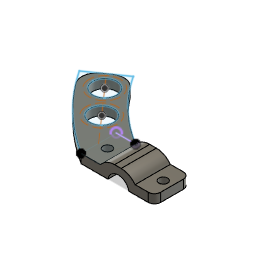
R1200GS Motorbike mirror button mount v3 (Autodesk Fusion 360 design; units mm, degrees)
Autodesk Fusion 360 part; units mm, degrees
sketch "Sketch1" plane through (0, 0, 0) normal (0, 0, 1) x (1, 0, 0)
  line L0 (0, 0) -> (15, 0) construction
  arc A0 (8.9159, -9.9997) -> (9.0729, 9.9997) centre (8.9986, 0) ccw
  line L1 (9.0729, 9.9997) -> (5.3447, 10.0008)
  arc A1 (5.3447, 10.0008) -> (5.3451, -10.0008) centre (5.3418, 0) ccw
  line L2 (5.3451, -10.0008) -> (8.9159, -9.9997)
  line L3 (0.0839, 1) -> (-13.6592, 1)
  line L4 (-13.6592, 1) -> (-13.6592, 6)
  line L5 (-13.6592, 6) -> (-2.6592, 6)
  line L6 (0.0839, 1) -> (27.9986, 1)
  line L7 (27.9986, 1) -> (27.9986, 6)
  line L8 (27.9986, 6) -> (16.9986, 6)
  circle A2 centre (7.5, 0) radius 6
  dimension "d4" = 5
  dimension "d6" = 5
  dimension "d7" = 1
  dimension "d8" = 1
  dimension "d52" = 11
  dimension "d53" = 11
  dimension "d122" = 12
  constraint horizontal L0
  constraint coincident L0.start origin
  constraint horizontal L3
  constraint perpendicular L3 L4
  constraint coincident A1 L5.end
  constraint perpendicular L4 L5
  constraint perpendicular L5 L7
  constraint coincident A0 L8.end
  constraint perpendicular L7 L8
  constraint tangent L1 A1
  constraint tangent A1 L2
  constraint midpoint L0 A2.centre
  constraint horizontal L6
  measures "d4" distance of L3.end L4.end
  measures "d6" distance of L6.end L7.end
  measures "d7" vertical distance of L0.start L3.start
  measures "d8" vertical distance of A0.centre L3.start
  measures "d52" distance of L7.end L8.end
  measures "d53" distance of L4.end L5.end
  measures "d122" diameter of A2
extrude "Extrude1" add sketch "Sketch1" along normal blind 20 contours A0 L1 A1 L3 L6 A2 | A0 L6 L7 L8 | A1 L3 L4 L5
hole "Hole1" at (-8.6592, 6, 10) direction (0, -1, 0) diameter 5 depth 5 tip angle 118
hole "Hole2" at (22.9986, 6, 10) direction (0, -1, 0) diameter 5 depth 5 tip angle 118
fillet "Fillet9" radius 3.5 2 edges at (27.9986, 3.5, 20) (27.9986, 3.5, 0)
sketch "Sketch7" plane through (0, 6, 0) normal (0, 1, 0) x (-1, 0, 0)
  circle A0 centre (8.6592, 10) radius 2.5
  line L0 (2.6592, 0) -> (13.6592, 0)
  line L1 (13.6592, 0) -> (13.6592, 20)
  line L2 (13.6592, 20) -> (2.6592, 20)
  line L3 (2.6592, 20) -> (2.6592, 0)
  line L4 (36.6932, -32.7022) -> (54.7147, -20.0838)
  line L5 (13.6592, 0) -> (2.6592, 0)
  circle A1 centre (39.0344, -18.8185) radius 6.8
  circle A2 centre (26.4668, -4.5455) radius 6.8
  line L6 (45.7039, -26.393) -> (13.6592, 10) construction
  circle A3 centre (39.0344, -18.8185) radius 8.75 construction
  circle A4 centre (26.4668, -4.5455) radius 8.75 construction
  arc A5 (54.7147, -20.0838) -> (13.6592, 20) centre (-60.9979, -97.5341) ccw
  arc A6 (36.6932, -32.7022) -> (2.6592, 0) centre (-53.2733, -92.2713) ccw
  dimension "d109" = 22
  dimension "d111" = 40
  dimension "d112" = 13.6
  dimension "d113" = 13.6
  dimension "d114" = 17.5
  dimension "d115" = 17.5
  constraint midpoint L4 L6.start
  constraint midpoint L1 L6.end
  constraint coincident A1.centre L6
  constraint coincident A2.centre L6
  constraint concentric A1 A3
  constraint concentric A2 A4
  constraint coincident L1.end L2.start
  constraint coincident L0.start L3.end
  measures "d109" distance of L4.start L4.end
  measures "d111" distance of L0.end L4.start
  measures "d112" diameter of A1
  measures "d113" diameter of A2
  measures "d114" diameter of A3
  measures "d115" diameter of A4
extrude "Extrude9" add sketch "Sketch7" against normal blind 5 contours L0 L1 L4 L5 A5 A6
fillet "Fillet8" radius 8.5 2 edges at (-54.7147, 3.5, -20.0838) (-36.6932, 3.5, -32.7022)
equation "d6 = d4"
equation "d8 = d7"
named bodies: "R1200GS front bar clamp"
